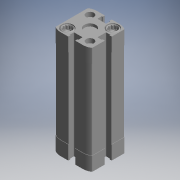
# Autodesk Inventor part: 536218 ADN-50-P---(Z)
Saved by Autodesk Inventor 2017.3 (Build 213256000, 256)
## iProperties
Part Number: 536218 ADN-50-P---(Z)
Material: Generic
Catalog Web Link: www.cadenas.de
Description: ADN-(Z)-Compact cylinder - Z
Vendor: FESTO
Document SubType Name: Modeling
Designer: partserver
Manufacturer: FESTO
Mass: 43.8204 g
Surface Area: 228.464 cm^2
Volume: 43.8204 cm^3
Density: 1 g/cm^3
Appearance: PSOLRGB-191-191-191
Category: PARTsolutions
Company: FESTO
Title: 536218 ADN-50-P---(Z)
Author: Cadenas PARTsolutions
Comments: Compact cylinder - Z
PSOL_IDENT_0: {$CADENAS_DATA\23d-libs\festo\parts\a\adn\parts\adn_zr.prj},211 {VTYP=3D},{NB=536218 ADN-50-P---(Z)}
PSOL_IDENT_1: ,{LINA=536218 ADN-50-P---(Z)},{NN=ADN-(Z)},{DATE=20.11.2019 12:35:12},{GEOMDATE=10.12.2018 13:24:47}
PSOL_IDENT_2: ,{VERSION=},{LINEID=8180},{WBVAR=HUB,DF,Q,S2S20,S1,R8,TT},{WBNUMERIC=HUB}  {NB=536218 ADN-50-P---(Z)
PSOL_IDENT_3: },{LINA=536218 ADN-50-P---(Z)},{KT=536218},{TNR=536218},{AUSF=ADN},{KDM=16},{BG=17.000},{VERS=1},{HU
PSOL_IDENT_4: BP=-},{HUB=50.00000},{HUB1=[1-300]},{HUB2=[1-200]},{HUB3=0},{THC='A','I'},{DF=P},{GA=A},{HUBL=variab
PSOL_IDENT_5: le},{HUBC=hubc error},{Q=-},{VAR1C='-','Q'},{S2S20=-},{VAR2C='-','S2','S20'},{VAR5C='-','S6'},{S1=-}
PSOL_IDENT_6: ,{R8=-},{R81='-'},{TT=-},{TT1='-'},{VAR6C='-'},{VAR7C='-','R3'},{HUBALG=[1-300]},{A=12.000},{A1=0.00
PSOL_IDENT_7: 0},{AF=10.000},{AF1=0.000},{AF2=10.000},{AF3=0.000},{B=0.000},{B1=0.000},{BG1=0.000},{D1=9.000},{D2=
PSOL_IDENT_8: 6.000},{D3=3.200},{D4=0.000},{D5=4.000},{D6=M3},{D7=3.000},{D8=3.200},{D9=4.500},{E=29.000},{EE=M5},
PSOL_IDENT_9: {EEN=5.000},{EE1=-},{J=11.000},{J1=2.600},{J11=2.6},{J2=0.000},{KF=8-36 UNF-2B},{KF1=-},{KF2=8-36 UN
PSOL_IDENT_10: F-2B},{KF3=-},{KK=10-32 UNF-2A},{KK1=-},{L1=1.500},{L2=35.000},{L3=2.100},{L4=3.500},{L5=0.000},{L6=
PSOL_IDENT_11: 46.000},{L7=14.000},{L8=3.000},{L9=1.500},{L10=0.000},{L11=0.000},{MF=6.000},{MM=8.000},{MM1=0.000},
PSOL_IDENT_12: {PL=6.000},{RT=M4},{RTN=4},{RTNK=3.242},{SF=9/32},{SF1=-},{SW=7.000},{TG=18.000},{VD=0.000},{VD1=0.0
PSOL_IDENT_13: 00},{WH=4.900},{WH1=0.000},{WL=3.700},{WL1=0.000},{Y1=0.300},{Y2=0.500},{ZJ=39.900},{ZM=44.800},{RU=
PSOL_IDENT_14: 18.600},{R1=9.550},{R2=0.600},{RA=0.000},{RB1=5.400},{RB2=6.800},{RT1=3.400},{DSK=6.000},{MDK=7.000}
PSOL_IDENT_15: ,{MK=4.000},{MT=2.000},{MS=3.000},{RUB=0.200},{KFN=4.000},{KFK=3.242},{B111=9.200},{B11=1.000},{B2=5
PSOL_IDENT_16: .000},{B3=8.500},{B4=3.500},{B5=3.000},{B6=6.000},{B7=17.000},{B8=4.000},{B9=6.000},{B10=7.200},{W=0
PSOL_IDENT_17: .400},{S=6.000},{LA=0.000},{LA1=0.000},{LA2=5.500},{LA3=6.700},{LA31=9.000},{LA4=0.000},{LA5=0.000},
PSOL_IDENT_18: {LA6=0.000},{RR=4.000},{LA7=0.000},{LA8=0.000},{LA9=0.000},{LA10=0.000},{ES=0.000},{SS=0.000},{TS=0.
PSOL_IDENT_19: 000},{WS=0.000},{DK=0.000},{KS=0.000},{QN=},{S2N=},{S1S20N=},{R8N=},{TTN=},{DFALG='P'}
NB: 536218 ADN-50-P---(Z)
NN: ADN-(Z)
NT: Compact cylinder - Z
NBSYN: $TNR. $AUSF.-$HUB.-$DF.$QN.$S2N.$S1S20N.$R8N.$TTN.---(Z)
LINA: 536218 ADN-50-P---(Z)
CATALOG: Festo
TNR: 536218
AUSF: ADN
KDM: 16
BG: 17
HUB: 50
DF: P
GA: A
Q: -
S2S20: -
S1: -
R8: -
TT: -
A: 12
A1: 0
AF: 10
AF1: 0
AF2: 10
AF3: 0
B: 0
B1: 0
BG1: 0
D1: 9
D2: 6
D3: 3.2
D4: 0
D5: 4
D6: M3
D7: 3
D8: 3.2
D9: 4.5
E: 29
EE: M5
EE1: -
J: 11
J1: 2.6
J2: 0
KF: 8-36 UNF-2B
KF1: -
KF2: 8-36 UNF-2B
KF3: -
KK: 10-32 UNF-2A
KK1: -
L1: 1.5
L2: 35
L3: 2.1
L4: 3.5
L5: 0
L6: 46
L7: 14
L8: 3
L9: 1.5
L10: 0
L11: 0
MF: 6
MM: 8
MM1: 0
PL: 6
RT: M4
RTNK: 3.242
SF: 9/32
SF1: -
SW: 7
TG: 18
VD: 0
VD1: 0
WH: 4.9
WH1: 0
WL: 3.7
WL1: 0
Y1: 0.3
Y2: 0.5
ZJ: 39.9
ZM: 44.8
RU: 18.6
R1: 9.55
R2: 0.6
RA: 0
DSK: 6
MDK: 7
MK: 4
MT: 2
MS: 3
RUB: 0.2
B111: 9.2
B11: 1
B2: 5
B3: 8.5
B4: 3.5
B5: 3
B6: 6
B7: 17
B8: 4
B9: 6
B10: 7.2
W: 0.4
S: 6
LA: 0
LA1: 0
LA2: 5.5
LA3: 6.7
LA31: 9
LA4: 0
LA5: 0
LA6: 0
RR: 4
LA7: 0
LA8: 0
LA9: 0
LA10: 0
ES: 0
SS: 0
TS: 0
WS: 0
DK: 0
KS: 0
SUPPLIER: FESTO
ARTICLENO: 536218 ADN-50-P---(Z)
BOMINFO: 536218 ADN-50-P---(Z)
CREATOR: CADENAS GmbH
Autodesk Inventor part; units mm, degrees
sketch "Skizze_1" plane through (0, 0, 0) normal (0, 0, 1) x (1, 0, 0)
  line L0 (-14.5, -3.1) -> (-14.5, -12.4395)
  arc A0 (-14.5, -12.4395) -> (-14.2285, -12.9416) centre (-13.9, -12.4395) ccw
  arc A1 (-14.2285, -12.9416) -> (-9, -14.5) centre (-9, -4.95) ccw
  line L1 (-9, -14.5) -> (-3.1, -14.5)
  arc A2 (-3.1, -14.5) -> (-2.7, -14.1) centre (-3.1, -14.1) ccw
  line L2 (-2.7, -14.1) -> (-2.7, -12.9)
  arc A3 (-2.7, -12.9) -> (-2.9, -12.7) centre (-2.9, -12.9) ccw
  line L3 (-2.9, -12.7) -> (-3.2, -12.7)
  arc A4 (-3.4, -12.5) -> (-3.2, -12.7) centre (-3.2, -12.5) ccw
  line L4 (-3.4, -12.5) -> (-3.4, -9.7)
  arc A5 (-3, -9.3) -> (-3.4, -9.7) centre (-3, -9.7) ccw
  line L5 (-3, -9.3) -> (3, -9.3)
  arc A6 (3.4, -9.7) -> (3, -9.3) centre (3, -9.7) ccw
  line L6 (3.4, -9.7) -> (3.4, -12.5)
  arc A7 (3.2, -12.7) -> (3.4, -12.5) centre (3.2, -12.5) ccw
  line L7 (3.2, -12.7) -> (2.9, -12.7)
  arc A8 (2.9, -12.7) -> (2.7, -12.9) centre (2.9, -12.9) ccw
  line L8 (2.7, -12.9) -> (2.7, -14.1)
  arc A9 (2.7, -14.1) -> (3.1, -14.5) centre (3.1, -14.1) ccw
  line L9 (3.1, -14.5) -> (9, -14.5)
  arc A10 (9, -14.5) -> (14.2285, -12.9416) centre (9, -4.95) ccw
  arc A11 (14.2285, -12.9416) -> (14.5, -12.4395) centre (13.9, -12.4395) ccw
  line L10 (14.5, -12.4395) -> (14.5, 12.4395)
  arc A12 (14.5, 12.4395) -> (14.2285, 12.9416) centre (13.9, 12.4395) ccw
  arc A13 (14.2285, 12.9416) -> (9, 14.5) centre (9, 4.95) ccw
  line L11 (9, 14.5) -> (3.1, 14.5)
  arc A14 (3.1, 14.5) -> (2.7, 14.1) centre (3.1, 14.1) ccw
  line L12 (2.7, 14.1) -> (2.7, 12.9)
  arc A15 (2.7, 12.9) -> (2.9, 12.7) centre (2.9, 12.9) ccw
  line L13 (2.9, 12.7) -> (3.2, 12.7)
  arc A16 (3.4, 12.5) -> (3.2, 12.7) centre (3.2, 12.5) ccw
  line L14 (3.4, 12.5) -> (3.4, 9.7)
  arc A17 (3, 9.3) -> (3.4, 9.7) centre (3, 9.7) ccw
  line L15 (3, 9.3) -> (-3, 9.3)
  arc A18 (-3.4, 9.7) -> (-3, 9.3) centre (-3, 9.7) ccw
  line L16 (-3.4, 9.7) -> (-3.4, 12.5)
  arc A19 (-3.2, 12.7) -> (-3.4, 12.5) centre (-3.2, 12.5) ccw
  line L17 (-3.2, 12.7) -> (-2.9, 12.7)
  arc A20 (-2.9, 12.7) -> (-2.7, 12.9) centre (-2.9, 12.9) ccw
  line L18 (-2.7, 12.9) -> (-2.7, 14.1)
  arc A21 (-2.7, 14.1) -> (-3.1, 14.5) centre (-3.1, 14.1) ccw
  line L19 (-3.1, 14.5) -> (-9, 14.5)
  arc A22 (-9, 14.5) -> (-14.2285, 12.9416) centre (-9, 4.95) ccw
  arc A23 (-14.2285, 12.9416) -> (-14.5, 12.4395) centre (-13.9, 12.4395) ccw
  line L20 (-14.5, 12.4395) -> (-14.5, 3.1)
  arc A24 (-14.5, 3.1) -> (-14.1, 2.7) centre (-14.1, 3.1) ccw
  line L21 (-14.1, 2.7) -> (-12.9, 2.7)
  arc A25 (-12.9, 2.7) -> (-12.7, 2.9) centre (-12.9, 2.9) ccw
  line L22 (-12.7, 2.9) -> (-12.7, 3.2)
  arc A26 (-12.5, 3.4) -> (-12.7, 3.2) centre (-12.5, 3.2) ccw
  line L23 (-12.5, 3.4) -> (-9.7, 3.4)
  arc A27 (-9.3, 3) -> (-9.7, 3.4) centre (-9.7, 3) ccw
  line L24 (-9.3, 3) -> (-9.3, -3)
  arc A28 (-9.7, -3.4) -> (-9.3, -3) centre (-9.7, -3) ccw
  line L25 (-9.7, -3.4) -> (-12.5, -3.4)
  arc A29 (-12.7, -3.2) -> (-12.5, -3.4) centre (-12.5, -3.2) ccw
  line L26 (-12.7, -3.2) -> (-12.7, -2.9)
  arc A30 (-12.7, -2.9) -> (-12.9, -2.7) centre (-12.9, -2.9) ccw
  line L27 (-12.9, -2.7) -> (-14.1, -2.7)
  arc A31 (-14.1, -2.7) -> (-14.5, -3.1) centre (-14.1, -3.1) ccw
  constraints: 64 point on circle, 56 end point, 32 centre point
extrude "Extrusion1" add sketch "Skizze_1" against normal blind 85
sketch "Sketch_111" plane through (0, 0, -11) normal (0, 0, 1) x (1, 0, 0)
  line L0 (-29, 29) -> (-29, -29)
  line L1 (-29, -29) -> (29, -29)
  line L2 (29, -29) -> (29, 29)
  line L3 (29, 29) -> (-29, 29)
  line L4 (-14.25, -3.1) -> (-14.25, -12.3472)
  arc A0 (-14.25, -12.3472) -> (-13.9617, -12.8599) centre (-13.65, -12.3472) ccw
  arc A1 (-13.9617, -12.8599) -> (-9, -14.25) centre (-9, -4.7) ccw
  line L5 (-9, -14.25) -> (-3.1, -14.25)
  arc A2 (-3.1, -14.25) -> (-2.7, -13.85) centre (-3.1, -13.85) ccw
  line L6 (-2.7, -13.85) -> (-2.7, -12.85)
  arc A3 (-2.7, -12.85) -> (-2.85, -12.7) centre (-2.85, -12.85) ccw
  line L7 (-2.85, -12.7) -> (-3.2, -12.7)
  arc A4 (-3.4, -12.5) -> (-3.2, -12.7) centre (-3.2, -12.5) ccw
  line L8 (-3.4, -12.5) -> (-3.4, -9.7)
  arc A5 (-3, -9.3) -> (-3.4, -9.7) centre (-3, -9.7) ccw
  line L9 (-3, -9.3) -> (3, -9.3)
  arc A6 (3.4, -9.7) -> (3, -9.3) centre (3, -9.7) ccw
  line L10 (3.4, -9.7) -> (3.4, -12.5)
  arc A7 (3.2, -12.7) -> (3.4, -12.5) centre (3.2, -12.5) ccw
  line L11 (3.2, -12.7) -> (2.85, -12.7)
  arc A8 (2.85, -12.7) -> (2.7, -12.85) centre (2.85, -12.85) ccw
  line L12 (2.7, -12.85) -> (2.7, -13.85)
  arc A9 (2.7, -13.85) -> (3.1, -14.25) centre (3.1, -13.85) ccw
  line L13 (3.1, -14.25) -> (9, -14.25)
  arc A10 (9, -14.25) -> (13.9617, -12.8599) centre (9, -4.7) ccw
  arc A11 (13.9617, -12.8599) -> (14.25, -12.3472) centre (13.65, -12.3472) ccw
  line L14 (14.25, -12.3472) -> (14.25, 12.3472)
  arc A12 (14.25, 12.3472) -> (13.9617, 12.8599) centre (13.65, 12.3472) ccw
  arc A13 (13.9617, 12.8599) -> (9, 14.25) centre (9, 4.7) ccw
  line L15 (9, 14.25) -> (3.1, 14.25)
  arc A14 (3.1, 14.25) -> (2.7, 13.85) centre (3.1, 13.85) ccw
  line L16 (2.7, 13.85) -> (2.7, 12.85)
  arc A15 (2.7, 12.85) -> (2.85, 12.7) centre (2.85, 12.85) ccw
  line L17 (2.85, 12.7) -> (3.2, 12.7)
  arc A16 (3.4, 12.5) -> (3.2, 12.7) centre (3.2, 12.5) ccw
  line L18 (3.4, 12.5) -> (3.4, 9.7)
  arc A17 (3, 9.3) -> (3.4, 9.7) centre (3, 9.7) ccw
  line L19 (3, 9.3) -> (-3, 9.3)
  arc A18 (-3.4, 9.7) -> (-3, 9.3) centre (-3, 9.7) ccw
  line L20 (-3.4, 9.7) -> (-3.4, 12.5)
  arc A19 (-3.2, 12.7) -> (-3.4, 12.5) centre (-3.2, 12.5) ccw
  line L21 (-3.2, 12.7) -> (-2.85, 12.7)
  arc A20 (-2.85, 12.7) -> (-2.7, 12.85) centre (-2.85, 12.85) ccw
  line L22 (-2.7, 12.85) -> (-2.7, 13.85)
  arc A21 (-2.7, 13.85) -> (-3.1, 14.25) centre (-3.1, 13.85) ccw
  line L23 (-3.1, 14.25) -> (-9, 14.25)
  arc A22 (-9, 14.25) -> (-13.9617, 12.8599) centre (-9, 4.7) ccw
  arc A23 (-13.9617, 12.8599) -> (-14.25, 12.3472) centre (-13.65, 12.3472) ccw
  line L24 (-14.25, 12.3472) -> (-14.25, 3.1)
  arc A24 (-14.25, 3.1) -> (-13.85, 2.7) centre (-13.85, 3.1) ccw
  line L25 (-13.85, 2.7) -> (-12.85, 2.7)
  arc A25 (-12.85, 2.7) -> (-12.7, 2.85) centre (-12.85, 2.85) ccw
  line L26 (-12.7, 2.85) -> (-12.7, 3.2)
  arc A26 (-12.5, 3.4) -> (-12.7, 3.2) centre (-12.5, 3.2) ccw
  line L27 (-12.5, 3.4) -> (-9.7, 3.4)
  arc A27 (-9.3, 3) -> (-9.7, 3.4) centre (-9.7, 3) ccw
  line L28 (-9.3, 3) -> (-9.3, -3)
  arc A28 (-9.7, -3.4) -> (-9.3, -3) centre (-9.7, -3) ccw
  line L29 (-9.7, -3.4) -> (-12.5, -3.4)
  arc A29 (-12.7, -3.2) -> (-12.5, -3.4) centre (-12.5, -3.2) ccw
  line L30 (-12.7, -3.2) -> (-12.7, -2.85)
  arc A30 (-12.7, -2.85) -> (-12.85, -2.7) centre (-12.85, -2.85) ccw
  line L31 (-12.85, -2.7) -> (-13.85, -2.7)
  arc A31 (-13.85, -2.7) -> (-14.25, -3.1) centre (-13.85, -3.1) ccw
  constraints: 64 end point, 64 point on circle, 32 centre point
extrude "Extrusion2" cut sketch "Sketch_111" against normal blind 63
sketch "Sketch3" plane through (14.5, -12.4395, 0) normal (1, 0, 0) x (0, 0, -1)
  point P0 (6, 9.8395)
hole "Hole1" at (14.5, -2.6, -6) direction (-1, 0, 0) diameter 4.134 depth 6.7 countersink diameter 5 countersink angle 90 thread size "M5x0.8" class "6H" standard "ISO Metric profile"
sketch "Sketch4" plane through (14.5, -12.4395, -85) normal (1, 0, 0) x (0, 0, -1)
  point P0 (-6, 15.0395)
hole "Hole2" at (14.5, 2.6, -79) direction (-1, 0, 0) diameter 4.134 depth 9 countersink diameter 5 countersink angle 90 thread size "M5x0.8" class "6H" standard "ISO Metric profile"
sketch "Skizze_5" plane through (0, 0, 0) normal (1, 0, 0) x (0, 1, 0)
  line L0 (0, -73) -> (0, 1)
  line L1 (0, 1) -> (4, 1)
  line L2 (4, 1) -> (4, -19)
  line L3 (4, -19) -> (8, -19)
  line L4 (8, -19) -> (8, -73)
  line L5 (8, -73) -> (0, -73)
  line L6 (0, -73) -> (0, 1)
  constraints: 14 end point
revolve "Revolution1" cut sketch "Skizze_5" angle 360 about axis through (0, 0, -73) along (0, 0, -1)
sketch "Sketch6" plane through (0, 0, -85) normal (0, 0, -1) x (-1, 0, 0)
  point P0 (0, 0)
hole "Hole3" at (0, 0, -85) direction (0, 0, 1) diameter 9 depth 2.1
sketch "Sketch7" plane through (0, 0, 0) normal (0, 0, 1) x (1, 0, 0)
  point P0 (9, 9)
hole "Hole4" at (9, 9, 0) direction (0, 0, -1) diameter 6 depth 17 counterbore diameter 9.2 counterbore depth 5
sketch "Sketch_27" plane through (9, 0, 0) normal (1, 0, 0) x (0, 0, -1)
  line L0 (17, 9) -> (0, 9)
  line L1 (0, 12.6) -> (1.0392, 12)
  line L2 (1.0392, 12) -> (3.5, 12)
  line L3 (3.5, 12) -> (3.5, 11)
  line L4 (3.5, 11) -> (3.879, 10.621)
  line L5 (3.879, 10.621) -> (17, 10.621)
  line L6 (17, 10.621) -> (17, 13)
  line L7 (17, 13) -> (5, 13)
  line L8 (5, 13) -> (5, 13.25)
  line L9 (5, 13.25) -> (0.4, 13.25)
  line L10 (0.4, 13.25) -> (0, 12.85)
  line L11 (0, 12.85) -> (0, 12.6)
  constraints: 24 end point
revolve "Revolution2" add sketch "Sketch_27" angle 360 about axis through (9, 9, -17) along (0, 0, -1)
thread "Thread1" size "M4x0.7" class "6H" standard "ISO Metric profile" full length
sketch "Sketch9" plane through (0, 0, -85) normal (0, 0, -1) x (-1, 0, 0)
  point P0 (-9, -9)
hole "Hole5" at (9, -9, -85) direction (0, 0, 1) diameter 6 depth 17 counterbore diameter 9.2 counterbore depth 5
sketch "Sketch_28" plane through (9, 0, 0) normal (1, 0, 0) x (0, 0, -1)
  line L0 (85, -9) -> (68, -9)
  line L1 (68, -5) -> (68, -7.379)
  line L2 (68, -7.379) -> (81.121, -7.379)
  line L3 (81.121, -7.379) -> (81.5, -7)
  line L4 (81.5, -7) -> (81.5, -6)
  line L5 (81.5, -6) -> (83.9608, -6)
  line L6 (83.9608, -6) -> (85, -5.4)
  line L7 (85, -5.4) -> (85, -5.15)
  line L8 (85, -5.15) -> (84.6, -4.75)
  line L9 (84.6, -4.75) -> (80, -4.75)
  line L10 (80, -4.75) -> (80, -5)
  line L11 (80, -5) -> (68, -5)
  constraints: 24 end point
revolve "Revolution3" add sketch "Sketch_28" angle 360 about axis through (9, -9, -85) along (0, 0, -1)
thread "Thread2" size "M4x0.7" class "6H" standard "ISO Metric profile" full length
sketch "Sketch11" plane through (0, 0, 0) normal (0, 0, 1) x (1, 0, 0)
  point P0 (-9, -9)
hole "Hole6" at (-9, -9, 0) direction (0, 0, -1) diameter 6 depth 17 counterbore diameter 9.2 counterbore depth 5
sketch "Sketch12" plane through (0, 0, -85) normal (0, 0, -1) x (-1, 0, 0)
  point P0 (9, 9)
hole "Hole7" at (-9, 9, -85) direction (0, 0, 1) diameter 6 depth 17 counterbore diameter 9.2 counterbore depth 5
sketch "Sketch_29" plane through (-9, 0, 0) normal (1, 0, 0) x (0, 0, -1)
  line L0 (17, -9) -> (0, -9)
  line L1 (0, -5.4) -> (1.0392, -6)
  line L2 (1.0392, -6) -> (3.5, -6)
  line L3 (3.5, -6) -> (3.5, -7)
  line L4 (3.5, -7) -> (3.879, -7.379)
  line L5 (3.879, -7.379) -> (17, -7.379)
  line L6 (17, -7.379) -> (17, -5)
  line L7 (17, -5) -> (5, -5)
  line L8 (5, -5) -> (5, -4.75)
  line L9 (5, -4.75) -> (0.4, -4.75)
  line L10 (0.4, -4.75) -> (0, -5.15)
  line L11 (0, -5.15) -> (0, -5.4)
  constraints: 24 end point
revolve "Revolution4" add sketch "Sketch_29" angle 360 about axis through (-9, -9, -17) along (0, 0, -1)
thread "Thread3" size "M4x0.7" class "6H" standard "ISO Metric profile" full length
sketch "Sketch_30" plane through (-9, 0, 0) normal (1, 0, 0) x (0, 0, -1)
  line L0 (85, 9) -> (68, 9)
  line L1 (68, 13) -> (68, 10.621)
  line L2 (68, 10.621) -> (81.121, 10.621)
  line L3 (81.121, 10.621) -> (81.5, 11)
  line L4 (81.5, 11) -> (81.5, 12)
  line L5 (81.5, 12) -> (83.9608, 12)
  line L6 (83.9608, 12) -> (85, 12.6)
  line L7 (85, 12.6) -> (85, 12.85)
  line L8 (85, 12.85) -> (84.6, 13.25)
  line L9 (84.6, 13.25) -> (80, 13.25)
  line L10 (80, 13.25) -> (80, 13)
  line L11 (80, 13) -> (68, 13)
  constraints: 24 end point
revolve "Revolution5" add sketch "Sketch_30" angle 360 about axis through (-9, 9, -85) along (0, 0, -1)
thread "Thread4" size "M4x0.7" class "6H" standard "ISO Metric profile" full length
sketch "Skizze_12" plane through (9, 0, 0) normal (1, 0, 0) x (0, 0, -1)
  line L0 (68, -9) -> (-0.1, -9)
  line L1 (-0.1, -9) -> (-0.1, -6)
  line L2 (-0.1, -6) -> (3.5, -6)
  line L3 (3.5, -6) -> (3.5, -7)
  line L4 (3.5, -7) -> (3.879, -7.379)
  line L5 (3.879, -7.379) -> (68, -7.379)
  line L6 (68, -7.379) -> (68, -9)
  line L7 (68, -9) -> (-0.1, -9)
  constraints: 16 end point
revolve "Revolution6" cut sketch "Skizze_12" angle 360 about axis through (9, -9, -68) along (0, 0, -1)
thread "Thread5" size "M4x0.7" class "6H" standard "ISO Metric profile" length 7.121
sketch "Sketch_123" plane through (9, 0, 0) normal (1, 0, 0) x (0, 0, -1)
  line L0 (68, -9) -> (11, -9)
  line L1 (11, -9) -> (11, -5)
  line L2 (11, -5) -> (68, -5)
  line L3 (68, -5) -> (68, -9)
  line L4 (68, -9) -> (11, -9)
  constraints: 10 end point
revolve "Revolution7" add sketch "Sketch_123" angle 360 about axis through (9, -9, -68) along (0, 0, -1)
sketch "Sketch17" plane through (9, -9, -68) normal (0, 0, -1) x (-1, 0, 0)
  point P0 (0, 0)
hole "Hole8" at (9, -9, -68) direction (0, 0, 1) diameter 4 depth 57
sketch "Sketch_3" plane through (9, 0, 0) normal (1, 0, 0) x (0, 0, -1)
  line L0 (85.1, 9) -> (42.5, 9)
  line L1 (42.5, 9) -> (42.5, 10.621)
  line L2 (42.5, 10.621) -> (81.121, 10.621)
  line L3 (81.121, 10.621) -> (81.5, 11)
  line L4 (81.5, 11) -> (81.5, 12)
  line L5 (81.5, 12) -> (85.1, 12)
  line L6 (85.1, 12) -> (85.1, 9)
  line L7 (85.1, 9) -> (42.5, 9)
  constraints: 16 end point
revolve "Revolution8" cut sketch "Sketch_3" angle 360 about axis through (9, 9, -85.1) along (0, 0, -1)
thread "Thread6" size "M4x0.7" class "6H" standard "ISO Metric profile" length 7.121
sketch "Sketch_117" plane through (9, 0, 0) normal (1, 0, 0) x (0, 0, -1)
  line L0 (74, 9) -> (17, 9)
  line L1 (17, 9) -> (17, 13)
  line L2 (17, 13) -> (74, 13)
  line L3 (74, 13) -> (74, 9)
  line L4 (74, 9) -> (17, 9)
  constraints: 10 end point
revolve "Revolution9" add sketch "Sketch_117" angle 360 about axis through (9, 9, -74) along (0, 0, -1)
sketch "Sketch20" plane through (9, 9, -74) normal (0, 0, -1) x (-1, 0, 0)
  point P0 (0, 0)
hole "Hole9" at (9, 9, -74) direction (0, 0, 1) diameter 4 depth 57
sketch "Skizze_13" plane through (-9, 0, 0) normal (1, 0, 0) x (0, 0, -1)
  line L0 (68, 9) -> (-0.1, 9)
  line L1 (-0.1, 9) -> (-0.1, 12)
  line L2 (-0.1, 12) -> (3.5, 12)
  line L3 (3.5, 12) -> (3.5, 11)
  line L4 (3.5, 11) -> (3.879, 10.621)
  line L5 (3.879, 10.621) -> (68, 10.621)
  line L6 (68, 10.621) -> (68, 9)
  line L7 (68, 9) -> (-0.1, 9)
  constraints: 16 end point
revolve "Revolution10" cut sketch "Skizze_13" angle 360 about axis through (-9, 9, -68) along (0, 0, -1)
thread "Thread7" size "M4x0.7" class "6H" standard "ISO Metric profile" length 7.121
sketch "Sketch_121" plane through (-9, 0, 0) normal (1, 0, 0) x (0, 0, -1)
  line L0 (68, 9) -> (11, 9)
  line L1 (11, 9) -> (11, 13)
  line L2 (11, 13) -> (68, 13)
  line L3 (68, 13) -> (68, 9)
  line L4 (68, 9) -> (11, 9)
  constraints: 10 end point
revolve "Revolution11" add sketch "Sketch_121" angle 360 about axis through (-9, 9, -68) along (0, 0, -1)
sketch "Sketch23" plane through (-9, 9, -68) normal (0, 0, -1) x (-1, 0, 0)
  point P0 (0, 0)
hole "Hole10" at (-9, 9, -68) direction (0, 0, 1) diameter 4 depth 57
sketch "Sketch_4" plane through (-9, 0, 0) normal (1, 0, 0) x (0, 0, -1)
  line L0 (85.1, -9) -> (42.5, -9)
  line L1 (42.5, -9) -> (42.5, -7.379)
  line L2 (42.5, -7.379) -> (81.121, -7.379)
  line L3 (81.121, -7.379) -> (81.5, -7)
  line L4 (81.5, -7) -> (81.5, -6)
  line L5 (81.5, -6) -> (85.1, -6)
  line L6 (85.1, -6) -> (85.1, -9)
  line L7 (85.1, -9) -> (42.5, -9)
  constraints: 16 end point
revolve "Revolution12" cut sketch "Sketch_4" angle 360 about axis through (-9, -9, -85.1) along (0, 0, -1)
thread "Thread8" size "M4x0.7" class "6H" standard "ISO Metric profile" length 7.121
sketch "Sketch_118" plane through (-9, 0, 0) normal (1, 0, 0) x (0, 0, -1)
  line L0 (74, -9) -> (17, -9)
  line L1 (17, -9) -> (17, -5)
  line L2 (17, -5) -> (74, -5)
  line L3 (74, -5) -> (74, -9)
  line L4 (74, -9) -> (17, -9)
  constraints: 10 end point
revolve "Revolution13" add sketch "Sketch_118" angle 360 about axis through (-9, -9, -74) along (0, 0, -1)
sketch "Sketch26" plane through (-9, -9, -74) normal (0, 0, -1) x (-1, 0, 0)
  point P0 (0, 0)
hole "Hole11" at (-9, -9, -74) direction (0, 0, 1) diameter 4 depth 57
sketch "Sketch_8" plane through (0, 0, 0) normal (0, 0, 1) x (1, 0, 0)
  line L0 (-12.4641, -9) -> (-12, -9.8038)
  line L1 (-12, -9.8038) -> (-12, -10.7321)
  line L2 (-12, -10.7321) -> (-11.1962, -11.1962)
  line L3 (-11.1962, -11.1962) -> (-10.7321, -12)
  line L4 (-10.7321, -12) -> (-9.8038, -12)
  line L5 (-9.8038, -12) -> (-9, -12.4641)
  line L6 (-9, -12.4641) -> (-8.1962, -12)
  line L7 (-8.1962, -12) -> (-7.2679, -12)
  line L8 (-7.2679, -12) -> (-6.8038, -11.1962)
  line L9 (-6.8038, -11.1962) -> (-6, -10.7321)
  line L10 (-6, -10.7321) -> (-6, -9.8038)
  line L11 (-6, -9.8038) -> (-5.5359, -9)
  line L12 (-5.5359, -9) -> (-6, -8.1962)
  line L13 (-6, -8.1962) -> (-6, -7.2679)
  line L14 (-6, -7.2679) -> (-6.8038, -6.8038)
  line L15 (-6.8038, -6.8038) -> (-7.2679, -6)
  line L16 (-7.2679, -6) -> (-8.1962, -6)
  line L17 (-8.1962, -6) -> (-9, -5.5359)
  line L18 (-9, -5.5359) -> (-9.8038, -6)
  line L19 (-9.8038, -6) -> (-10.7321, -6)
  line L20 (-10.7321, -6) -> (-11.1962, -6.8038)
  line L21 (-11.1962, -6.8038) -> (-12, -7.2679)
  line L22 (-12, -7.2679) -> (-12, -8.1962)
  line L23 (-12, -8.1962) -> (-12.4641, -9)
  constraints: 48 end point
extrude "Extrusion3" cut sketch "Sketch_8" against normal blind 3
sketch "Sketch_7" plane through (0, 0, 0) normal (0, 0, 1) x (1, 0, 0)
  line L0 (5.5359, 9) -> (6, 8.1962)
  line L1 (6, 8.1962) -> (6, 7.2679)
  line L2 (6, 7.2679) -> (6.8038, 6.8038)
  line L3 (6.8038, 6.8038) -> (7.2679, 6)
  line L4 (7.2679, 6) -> (8.1962, 6)
  line L5 (8.1962, 6) -> (9, 5.5359)
  line L6 (9, 5.5359) -> (9.8038, 6)
  line L7 (9.8038, 6) -> (10.7321, 6)
  line L8 (10.7321, 6) -> (11.1962, 6.8038)
  line L9 (11.1962, 6.8038) -> (12, 7.2679)
  line L10 (12, 7.2679) -> (12, 8.1962)
  line L11 (12, 8.1962) -> (12.4641, 9)
  line L12 (12.4641, 9) -> (12, 9.8038)
  line L13 (12, 9.8038) -> (12, 10.7321)
  line L14 (12, 10.7321) -> (11.1962, 11.1962)
  line L15 (11.1962, 11.1962) -> (10.7321, 12)
  line L16 (10.7321, 12) -> (9.8038, 12)
  line L17 (9.8038, 12) -> (9, 12.4641)
  line L18 (9, 12.4641) -> (8.1962, 12)
  line L19 (8.1962, 12) -> (7.2679, 12)
  line L20 (7.2679, 12) -> (6.8038, 11.1962)
  line L21 (6.8038, 11.1962) -> (6, 10.7321)
  line L22 (6, 10.7321) -> (6, 9.8038)
  line L23 (6, 9.8038) -> (5.5359, 9)
  constraints: 48 end point
extrude "Extrusion4" cut sketch "Sketch_7" against normal blind 3
sketch "Sketch_9" plane through (0, 0, -85) normal (0, 0, 1) x (1, 0, 0)
  line L0 (-12.4641, 9) -> (-12, 8.1962)
  line L1 (-12, 8.1962) -> (-12, 7.2679)
  line L2 (-12, 7.2679) -> (-11.1962, 6.8038)
  line L3 (-11.1962, 6.8038) -> (-10.7321, 6)
  line L4 (-10.7321, 6) -> (-9.8038, 6)
  line L5 (-9.8038, 6) -> (-9, 5.5359)
  line L6 (-9, 5.5359) -> (-8.1962, 6)
  line L7 (-8.1962, 6) -> (-7.2679, 6)
  line L8 (-7.2679, 6) -> (-6.8038, 6.8038)
  line L9 (-6.8038, 6.8038) -> (-6, 7.2679)
  line L10 (-6, 7.2679) -> (-6, 8.1962)
  line L11 (-6, 8.1962) -> (-5.5359, 9)
  line L12 (-5.5359, 9) -> (-6, 9.8038)
  line L13 (-6, 9.8038) -> (-6, 10.7321)
  line L14 (-6, 10.7321) -> (-6.8038, 11.1962)
  line L15 (-6.8038, 11.1962) -> (-7.2679, 12)
  line L16 (-7.2679, 12) -> (-8.1962, 12)
  line L17 (-8.1962, 12) -> (-9, 12.4641)
  line L18 (-9, 12.4641) -> (-9.8038, 12)
  line L19 (-9.8038, 12) -> (-10.7321, 12)
  line L20 (-10.7321, 12) -> (-11.1962, 11.1962)
  line L21 (-11.1962, 11.1962) -> (-12, 10.7321)
  line L22 (-12, 10.7321) -> (-12, 9.8038)
  line L23 (-12, 9.8038) -> (-12.4641, 9)
  constraints: 48 end point
extrude "Extrusion5" cut sketch "Sketch_9" along normal blind 3
sketch "Sketch_10" plane through (0, 0, -85) normal (0, 0, 1) x (1, 0, 0)
  line L0 (5.5359, -9) -> (6, -9.8038)
  line L1 (6, -9.8038) -> (6, -10.7321)
  line L2 (6, -10.7321) -> (6.8038, -11.1962)
  line L3 (6.8038, -11.1962) -> (7.2679, -12)
  line L4 (7.2679, -12) -> (8.1962, -12)
  line L5 (8.1962, -12) -> (9, -12.4641)
  line L6 (9, -12.4641) -> (9.8038, -12)
  line L7 (9.8038, -12) -> (10.7321, -12)
  line L8 (10.7321, -12) -> (11.1962, -11.1962)
  line L9 (11.1962, -11.1962) -> (12, -10.7321)
  line L10 (12, -10.7321) -> (12, -9.8038)
  line L11 (12, -9.8038) -> (12.4641, -9)
  line L12 (12.4641, -9) -> (12, -8.1962)
  line L13 (12, -8.1962) -> (12, -7.2679)
  line L14 (12, -7.2679) -> (11.1962, -6.8038)
  line L15 (11.1962, -6.8038) -> (10.7321, -6)
  line L16 (10.7321, -6) -> (9.8038, -6)
  line L17 (9.8038, -6) -> (9, -5.5359)
  line L18 (9, -5.5359) -> (8.1962, -6)
  line L19 (8.1962, -6) -> (7.2679, -6)
  line L20 (7.2679, -6) -> (6.8038, -6.8038)
  line L21 (6.8038, -6.8038) -> (6, -7.2679)
  line L22 (6, -7.2679) -> (6, -8.1962)
  line L23 (6, -8.1962) -> (5.5359, -9)
  constraints: 48 end point
extrude "Extrusion6" cut sketch "Sketch_10" along normal blind 3
ref_plane "CYLINDER_XY" through (0, 0, -73) normal (0, 0, 1) x (1, 0, 0)
ref_plane "CYLINDER_YZ" through (0, 0, -73) normal (1, 0, 0) x (0, 1, 0)
ref_plane "CYLINDER_ZX" through (0, 0, -73) normal (0, 1, 0) x (0, 0, 1)
ref_plane "FDT_FRONT_XY" through (0, 0, 0) normal (0, 0, 1) x (0, -1, 0)
ref_plane "FDT_FRONT_YZ" through (0, 0, 0) normal (0, -1, 0) x (1, 0, 0)
ref_plane "FDT_FRONT_ZX" through (0, 0, 0) normal (1, 0, 0) x (0, 0, 1)
ref_plane "FDT_QSFRONT_XY" through (14.5, -2.6, -6) normal (1, 0, 0) x (0, -1, 0)
ref_plane "FDT_QSFRONT_YZ" through (14.5, -2.6, -6) normal (0, -1, 0) x (0, 0, -1)
ref_plane "FDT_QSFRONT_ZX" through (14.5, -2.6, -6) normal (0, 0, -1) x (1, 0, 0)
ref_plane "FDT_QSREAR_XY" through (14.5, 2.6, -79) normal (1, 0, 0) x (0, -1, 0)
ref_plane "FDT_QSREAR_YZ" through (14.5, 2.6, -79) normal (0, -1, 0) x (0, 0, -1)
ref_plane "FDT_QSREAR_ZX" through (14.5, 2.6, -79) normal (0, 0, -1) x (1, 0, 0)
ref_plane "FDT_REAR_XY" through (0, 0, -85) normal (0, 0, 1) x (0, -1, 0)
ref_plane "FDT_REAR_YZ" through (0, 0, -85) normal (0, -1, 0) x (1, 0, 0)
ref_plane "FDT_REAR_ZX" through (0, 0, -85) normal (1, 0, 0) x (0, 0, 1)
ref_plane "FDT_SLOT3_1_XY" through (0, 9.3, -42.5) normal (0, 1, 0) x (1, 0, 0)
ref_plane "FDT_SLOT3_1_YZ" through (0, 9.3, -42.5) normal (1, 0, 0) x (0, 0, -1)
ref_plane "FDT_SLOT3_1_ZX" through (0, 9.3, -42.5) normal (0, 0, -1) x (0, 1, 0)
ref_plane "FDT_SLOT5_1_XY" through (-9.3, 0, -42.5) normal (-1, 0, 0) x (0, 1, 0)
ref_plane "FDT_SLOT5_1_YZ" through (-9.3, 0, -42.5) normal (0, 1, 0) x (0, 0, -1)
ref_plane "FDT_SLOT5_1_ZX" through (-9.3, 0, -42.5) normal (0, 0, -1) x (-1, 0, 0)
ref_plane "FDT_SLOT7_1_XY" through (0, -9.3, -42.5) normal (0, -1, 0) x (-1, 0, 0)
ref_plane "FDT_SLOT7_1_YZ" through (0, -9.3, -42.5) normal (-1, 0, 0) x (0, 0, -1)
ref_plane "FDT_SLOT7_1_ZX" through (0, -9.3, -42.5) normal (0, 0, -1) x (0, -1, 0)
ref_plane "TO_DUMMY_XY" through (0, 0, 0) normal (0, 0, 1) x (1, 0, 0)
ref_plane "TO_DUMMY_YZ" through (0, 0, 0) normal (1, 0, 0) x (0, 1, 0)
ref_plane "TO_DUMMY_ZX" through (0, 0, 0) normal (0, 1, 0) x (0, 0, 1)
body "Solid1"
